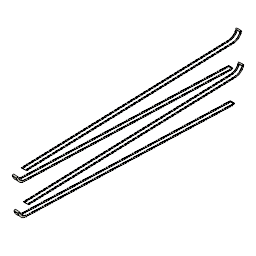
ball ramp (Autodesk Fusion 360 design; units mm, degrees)
part number: 2026-03-27-14-22-18-782
Autodesk Fusion 360 part; units mm, degrees
sketch "Sketch1" plane through (0, 0, 0) normal (1, 0, 0) x (0, 1, 0)
  line L0 (-50.8, 50.8) -> (-48.1587, 42.8761)
  line L1 (-6.3093, 11.6394) -> (1167.7292, -27.5278)
  arc A0 (-48.1587, 42.8761) -> (-6.3093, 11.6394) centre (-4.7849, 57.334) ccw
  line L2 (-50.8, 50.8) -> (-48.1587, 42.8761)
  arc A1 (-48.1587, 42.8761) -> (-6.3093, 11.6394) centre (-4.7849, 57.334) ccw
  arc A2 (-41.8087, 49.2261) -> (0.0407, 17.9894) centre (1.5651, 63.684) ccw
  line L3 (-44.45, 57.15) -> (-41.8087, 49.2261)
  line L4 (0.0407, 17.9894) -> (1174.0792, -21.1778)
  line L5 (-50.8, 50.8) -> (-44.45, 57.15)
  line L6 (1174.0792, -21.1778) -> (1167.7292, -27.5278)
extrude "Extrude1" add sketch "Sketch1" along normal blind 25.4 makes body 1
sketch "Sketch2" plane through (0, 0, 0) normal (0, 0, 1) x (1, 0, 0)
  line L0 (2.54, 1170.94) -> (22.86, 1170.94)
  line L1 (22.86, 1170.94) -> (22.86, -40.64)
  line L2 (22.86, -40.64) -> (2.54, -40.64)
  line L3 (2.54, -40.64) -> (2.54, 1170.94)
  constraint horizontal L0
  constraint vertical L1
  constraint horizontal L2
  constraint vertical L3
extrude "Extrude2" cut sketch "Sketch2" against normal blind 25.4 bodies 1
extrude "Extrude3" cut 1 faces at (9.3133, 1147.8878, -25.4) along direction (0, 0, -1) blind 12.7 on bodies 1 bodies 1
sketch "Sketch3" plane through (0, 0.5995, 17.9708) normal (0, 0.033343, 0.999444) x (-1, 0, 0)
  line L0 (-22.86, -1170.9916) -> (-22.86, -538.975)
  line L1 (-22.86, -538.975) -> (-2.54, -538.975)
  line L2 (-2.54, -538.975) -> (-2.54, -1170.9916)
  line L3 (-2.54, -1170.9916) -> (-22.86, -1170.9916)
  line L4 (0, -1174.1325) -> (0, 0.5591)
  line L5 (0, 0.5591) -> (-25.4, 0.5591)
  line L6 (-25.4, 0.5591) -> (-25.4, -1174.1325)
  line L7 (-25.4, -1174.1325) -> (0, -1174.1325)
  line L8 (-2.54, -538.975) -> (-22.86, -538.975)
  line L9 (-22.86, -538.975) -> (-22.86, 0.5591)
  line L10 (-22.86, 0.5591) -> (-2.54, 0.5591)
  line L11 (-2.54, 0.5591) -> (-2.54, -538.975)
  constraint horizontal L8
  constraint vertical L9
  constraint horizontal L10
  constraint vertical L11
  constraint coincident L1.end L2.start
extrude "Extrude4" cut sketch "Sketch3" against normal blind 25.4 contours L1 L5 L8 L9 L10 L11 bodies 1
sketch "Sketch4" plane through (0, 0, 0) normal (0, 1, 0) x (1, 0, 0)
  line L0 (22.86, -17.78) -> (2.54, -17.78)
  line L1 (2.54, -17.78) -> (2.54, -48.26)
  line L2 (2.54, -48.26) -> (22.86, -48.26)
  line L3 (22.86, -48.26) -> (22.86, -17.78)
  constraint horizontal L0
  constraint vertical L1
  constraint horizontal L2
  constraint vertical L3
extrude "Extrude5" cut sketch "Sketch4" against normal blind 76.2 bodies 1
sketch "Sketch5" plane through (0, 0, 17.78) normal (0, 0, 1) x (-1, 0, 0)
  line L0 (-2.54, 27.7152) -> (-22.86, 27.7152)
  line L1 (-22.86, 27.7152) -> (-22.86, 0)
  line L2 (-22.86, 0) -> (-2.54, 0)
  line L3 (-2.54, 0) -> (-2.54, 27.7152)
  line L4 (-22.86, 27.7152) -> (-2.54, 27.7152)
  line L5 (-2.54, 27.7152) -> (-2.54, 0)
  line L6 (-2.54, 0) -> (-22.86, 0)
  line L7 (-22.86, 0) -> (-22.86, 27.7152)
  constraint horizontal L4
  constraint vertical L5
  constraint horizontal L6
  constraint vertical L7
  constraint coincident L2.end L3.start
  constraint coincident L0.end L1.start
extrude "Extrude6" cut sketch "Sketch5" against normal blind 50.8 bodies 1
sketch "Sketch6" plane through (0, 0, 0) normal (0, 0, 1) x (1, 0, 0)
  line L0 (2.54, 0) -> (22.7468, 0)
  line L1 (22.7468, 0) -> (22.7468, -0.7767)
  line L2 (22.7468, -0.7767) -> (2.54, -0.7767)
  line L3 (2.54, -0.7767) -> (2.54, 0)
  constraint horizontal L0
  constraint vertical L1
  constraint horizontal L2
  constraint vertical L3
extrude "Extrude8" add 1 faces at (9.3133, 0, 17.5838) along direction (0, -1, 0) blind 2.54 on bodies 1 bodies 1
extrude "Extrude9" cut 1 faces at (16.0867, -0.8467, 17.9908) along direction (0, 0, -1) blind 11.43 on bodies 1 bodies 1
extrude "Extrude10" add 1 faces at (9.3133, 0, 17.5838) along direction (0, -1, 0) blind 27.94 on bodies 1 bodies 1
extrude "Extrude11" cut 1 faces at (16.0867, -9.3133, 17.9908) along direction (0, 0, -1) blind 3.81 on bodies 1 bodies 1
delete_face "DeleteFace1" 1 faces at (9.3133, 0, 17.5838) on bodies 1
copy_body "CopyPasteBodies1" bodies 1 makes body 2
move_body "Move1" bodies 2 to x (-1, 0, 0) y (0, -1, 0) z (0, 0, 1) at (-55.5923, -85.9135, 71.2788)
move_body "Move2" bodies 2 to x (1, 0, 0) y (0, 1, 0) z (0, 0, 1) at (79.5366, 1261.74, 18.7826)
copy_body "CopyPasteBodies2" bodies 1 2 makes body 3 makes body 4
move_body "Move3" bodies 3 4 to x (1, 0, 0) y (0, 1, 0) z (0, 0, 1) at (-0.0572, -10.8207, 171.5712)
move_body "Move4" bodies 3 to x (1, 0, 0) y (0, 1, 0) z (0, 0, 1) at (0, 1.2045, 6.0225)
move_body "Move5" bodies 2 to x (1, 0, 0) y (0, 1, 0) z (0, 0, 1) at (0, -15.6585, -1.2045)
move_body "Move6" bodies 2 to x (1, 0, 0) y (0, 1, 0) z (0, 0, 1) at (0, 16.863, 0)
